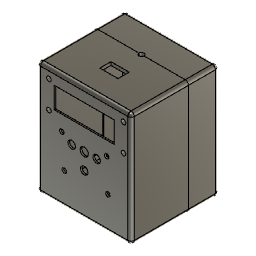
alarmClock (Autodesk Fusion 360 design; units mm, degrees)
Autodesk Fusion 360 part; units mm, degrees
sketch "Sketch1" plane through (0, 0, 0) normal (0, 0, 1) x (1, 0, 0)
  line L0 (35, 32.5) -> (-35, 32.5)
  line L1 (-35, 32.5) -> (-35, -32.5)
  line L2 (-35, -32.5) -> (35, -32.5)
  line L3 (35, -32.5) -> (35, 32.5)
  line L4 (35, 32.5) -> (-35, -32.5) construction
  line L5 (-35, 32.5) -> (35, -32.5) construction
  dimension "d6" = 70
  dimension "d7" = 65
  constraint horizontal L0
  constraint perpendicular L0 L1
  constraint parallel L0 L2
  constraint parallel L1 L3
  constraint coincident L4 origin
  constraint coincident L5 origin
  measures "d6" distance of L1.end L2.end
  measures "d7" distance of L0.end L1.end
extrude "Extrude1" add sketch "Sketch1" along normal blind 86 makes body 1
shell "Shell1" thickness 2.6 outward yes removed faces 0 bodies 1
sketch "Sketch2" plane through (0, 32.5, 0) normal (0, -1, 0) x (1, 0, 0)
  line L0 (-35, 0) -> (35, 0)
  line L1 (35, 0) -> (35, 86)
  line L2 (35, 86) -> (-35, 86)
  line L3 (-35, 86) -> (-35, 0)
  line L4 (28.1, 0) -> (19.9, 0)
  line L5 (19.9, 0) -> (19.9, 4.4)
  line L6 (19.9, 4.4) -> (28.1, 4.4)
  line L7 (28.1, 4.4) -> (28.1, 0)
  line L8 (24, 4.4) -> (24, 0) construction
  dimension "d11" = 8.2
  dimension "d12" = 4.4
  dimension "d13" = 11
  constraint horizontal L4
  constraint vertical L5
  constraint horizontal L6
  constraint vertical L7
  constraint coincident L0 L4.start
  constraint midpoint L6 L8.start
  constraint midpoint L4 L8.end
  measures "d11" distance of L5 L7
  measures "d12" distance of L4 L6
  measures "d13" distance of L1 L8
extrude "Extrude2" cut sketch "Sketch2" against normal up to surface (2.6 mm away) contours L0 L4 L5 L6 L7 bodies 1
sketch "Sketch3" plane through (0, 0, 0) normal (0, 0, 1) x (-1, 0, 0)
  line L0 (-35, 32.5) -> (-35, -32.5)
  line L1 (-35, -32.5) -> (-28.1, -32.5)
  line L2 (-28.1, -32.5) -> (-28.1, -35.1)
  line L3 (-28.1, -35.1) -> (-19.9, -35.1)
  line L4 (-19.9, -35.1) -> (-19.9, -32.5)
  line L5 (-19.9, -32.5) -> (35, -32.5)
  line L6 (35, -32.5) -> (35, 32.5)
  line L7 (35, 32.5) -> (-35, 32.5)
  line L8 (-24, -35.1) -> (-24, 32.5) construction
  line L9 (-16.6, -30.5) -> (-31.4, -30.5) construction
  line L10 (-31.4, -30.5) -> (-31.4, 10) construction
  line L11 (-31.4, 10) -> (-16.6, 10) construction
  line L12 (-16.6, 10) -> (-16.6, -30.5) construction
  circle A0 centre (-16.6, 10) radius 0.605
  circle A1 centre (-31.4, 10) radius 0.605
  circle A2 centre (-31.4, -30.5) radius 0.605
  circle A3 centre (-16.6, -30.5) radius 0.605
  line L13 (-31.4, 11.9) -> (-16.6, 11.9)
  line L14 (-16.6, 11.9) -> (-31.4, 11.9)
  line L15 (-31.4, 11.9) -> (-31.4, 13.3)
  line L16 (-31.4, 13.3) -> (-16.6, 13.3)
  line L17 (-16.6, 13.3) -> (-16.6, 11.9)
  line L18 (30.7, -26.5) -> (13, -26.5) construction
  line L19 (13, -26.5) -> (13, -0.8) construction
  line L20 (13, -0.8) -> (30.7, -0.8) construction
  line L21 (30.7, -0.8) -> (30.7, -26.5) construction
  circle A4 centre (13, -26.5) radius 1.5
  circle A5 centre (30.7, -26.5) radius 1.5
  circle A6 centre (30.7, -0.8) radius 1.5
  circle A7 centre (13, -0.8) radius 1.5
  line L22 (35, -10.8333) -> (-35, -10.8333) construction
  point P0 (-24, -30.5)
  dimension "d16" = 40.5
  dimension "d17" = 14.8
  dimension "d18" = 2
  dimension "d19" = 1.21
  dimension "d20" = 1.21
  dimension "d21" = 1.21
  dimension "d22" = 1.21
  dimension "d25" = -1.9
  dimension "d26" = 1.4
  dimension "d29" = 22
  dimension "d30" = 6
  dimension "d31" = 17.7
  dimension "d32" = 25.7
  dimension "d33" = 3
  dimension "d34" = 3
  dimension "d35" = 3
  dimension "d36" = 3
  dimension "d93" = 21.6667
  constraint midpoint L3 L8.start
  constraint coincident L7 L8.end
  constraint perpendicular L7 L8
  constraint horizontal L9
  constraint vertical L10
  constraint horizontal L11
  constraint vertical L12
  constraint midpoint L9 P0
  constraint coincident L8 P0
  constraint coincident L11.end L12.start
  constraint coincident L10.end L11.start
  constraint coincident L9.end L10.start
  constraint coincident L9.start L12.end
  constraint horizontal L14
  constraint vertical L15
  constraint horizontal L16
  constraint vertical L17
  constraint coincident L13.start L15
  constraint horizontal L18
  constraint vertical L19
  constraint horizontal L20
  constraint vertical L21
  constraint coincident L18.end L19.start
  constraint coincident L18.start L21.end
  constraint coincident L20.end L21.start
  constraint coincident L19.end L20.start
  constraint coincident L6 L22.start
  constraint coincident L0 L22.end
  constraint perpendicular L0 L22
  measures "d16" distance of L9 L11
  measures "d17" distance of L10 L12
  measures "d18" distance of L5 L9
  measures "d19" diameter of A0
  measures "d20" diameter of A1
  measures "d21" diameter of A2
  measures "d22" diameter of A3
  measures "d26" distance of L13 L16
  measures "d29" distance of L6 L19
  measures "d30" distance of L5 L18
  measures "d31" distance of L19 L21
  measures "d32" distance of L18 L20
  measures "d33" diameter of A7
  measures "d34" diameter of A6
  measures "d35" diameter of A5
  measures "d36" diameter of A4
  measures "d93" distance of L5 L22
extrude "Extrude5" cut sketch "Sketch3" against normal up to surface (2.6 mm away) contours A4 | A5 | A6 | A7 bodies 1
extrude "Extrude3" cut sketch "Sketch3" against normal up to surface (2.6 mm away) contours A0 | A1 | A2 | A3 bodies 1
extrude "Extrude4" add sketch "Sketch3" along normal blind 7.2 contours L13 L14 L15 L16 L17 bodies 1
chamfer "Chamfer2" distance 7 angle 45 1 edges at (24, -13.3, 0) on bodies 1
sketch "Sketch4" plane through (0, -32.5, 0) normal (0, 1, 0) x (-1, 0, 0)
  line L0 (-35, 0) -> (35, 0)
  line L1 (35, 0) -> (35, 86)
  line L2 (35, 86) -> (-35, 86)
  line L3 (-35, 86) -> (-35, 0)
  line L4 (0, 86) -> (0, 0) construction
  circle A0 centre (0, 31) radius 3
  circle A1 centre (0, 44) radius 3.3
  line L5 (-35, 44) -> (35, 44) construction
  circle A2 centre (10, 44) radius 3
  circle A3 centre (-10, 44) radius 3
  line L6 (10, 44) -> (18, 44) construction
  line L7 (18, 44) -> (18, 50) construction
  line L8 (18, 50) -> (10, 50) construction
  line L9 (10, 50) -> (10, 44) construction
  line L10 (-10, 44) -> (-18, 44) construction
  line L11 (-18, 44) -> (-18, 49) construction
  line L12 (-18, 49) -> (-10, 49) construction
  line L13 (-10, 49) -> (-10, 44) construction
  line L14 (18, 50) -> (19, 50) construction
  line L15 (19, 50) -> (19, 24) construction
  line L16 (19, 24) -> (18, 24) construction
  line L17 (18, 24) -> (18, 50) construction
  line L18 (-18, 49) -> (-16, 49) construction
  line L19 (-16, 49) -> (-16, 23) construction
  line L20 (-16, 23) -> (-18, 23) construction
  line L21 (-18, 23) -> (-18, 49) construction
  circle A4 centre (-16, 23) radius 1.8 construction
  circle A5 centre (19, 24) radius 1.8 construction
  circle A6 centre (18, 50) radius 1.8 construction
  circle A7 centre (-18, 49) radius 1.8 construction
  line L22 (26.1, 59.2) -> (-26.1, 59.2)
  line L23 (-26.1, 59.2) -> (-26.1, 80.2)
  line L24 (-26.1, 80.2) -> (26.1, 80.2)
  line L25 (26.1, 80.2) -> (26.1, 59.2)
  line L26 (26.1, 59.2) -> (-26.1, 80.2) construction
  line L27 (-26.1, 59.2) -> (26.1, 80.2) construction
  line L28 (-24.1, 78.2) -> (24.1, 78.2)
  line L29 (24.1, 78.2) -> (24.1, 61.2)
  line L30 (24.1, 61.2) -> (-24.1, 61.2)
  line L31 (-24.1, 61.2) -> (-24.1, 78.2)
  line L32 (31.5, 80.5) -> (31.5, 58.8) construction
  line L33 (31.5, 80.5) -> (31.5, 58.8) construction
  line L34 (31.5, 58.8) -> (-28.3, 58.8) construction
  line L35 (-28.3, 58.8) -> (-28.3, 80.5) construction
  line L36 (-28.3, 80.5) -> (31.5, 80.5) construction
  circle A8 centre (31.5, 80.5) radius 1.85 construction
  circle A9 centre (31.5, 58.8) radius 1.85 construction
  circle A10 centre (-28.3, 80.5) radius 1.85 construction
  circle A11 centre (-28.3, 58.8) radius 1.85 construction
  circle A12 centre (18, 49) radius 1.8
  circle A13 centre (16, 23) radius 1.8
  circle A14 centre (-18, 50) radius 1.8
  circle A15 centre (-19, 24) radius 1.8
  circle A16 centre (28.3, 58.8) radius 1.85
  circle A17 centre (28.3, 80.5) radius 1.85
  circle A18 centre (-31.5, 80.5) radius 1.85
  circle A19 centre (-31.5, 58.8) radius 1.85
  line L37 (28, 55) -> (-29, 55)
  line L38 (-29, 55) -> (-29, 18)
  line L39 (-29, 18) -> (28, 18)
  line L40 (28, 18) -> (28, 55)
  point P0 (0, 69.7)
  dimension "d39" = 31
  dimension "d40" = 13
  dimension "d41" = 10
  dimension "d42" = 10
  dimension "d43" = 6
  dimension "d44" = 6
  dimension "d45" = 6
  dimension "d46" = 6.6
  dimension "d47" = 8
  dimension "d48" = 6
  dimension "d49" = 8
  dimension "d50" = 5
  dimension "d51" = 26
  dimension "d52" = 1
  dimension "d53" = 2
  dimension "d54" = 26
  dimension "d55" = 3.6
  dimension "d56" = 3.6
  dimension "d57" = 3.6
  dimension "d58" = 3.6
  dimension "d59" = 52.2
  dimension "d60" = 21
  dimension "d61" = 15.2
  dimension "d62" = 2
  dimension "d63" = 5.4
  dimension "d64" = 0.3
  dimension "d65" = 0.4
  dimension "d66" = 2.2
  dimension "d67" = 3.7
  dimension "d68" = 3.7
  dimension "d69" = 3.7
  dimension "d70" = 3.7
  dimension "d125" = 5
  dimension "d126" = 10
  dimension "d127" = 10
  dimension "d128" = 5
  constraint midpoint L2 L4.start
  constraint coincident L4.end origin
  constraint coincident L4 A0.centre
  constraint coincident L4 A1.centre
  constraint coincident L3 L5.start
  constraint coincident L1 L5.end
  constraint perpendicular L1 L5
  constraint coincident A1.centre L5
  constraint coincident L5 A2.centre
  constraint coincident L5 A3.centre
  constraint horizontal L6
  constraint vertical L7
  constraint horizontal L8
  constraint vertical L9
  constraint coincident A2.centre L6.start
  constraint horizontal L10
  constraint vertical L11
  constraint horizontal L12
  constraint vertical L13
  constraint coincident A3.centre L10.start
  constraint horizontal L14
  constraint vertical L15
  constraint horizontal L16
  constraint vertical L17
  constraint horizontal L18
  constraint vertical L19
  constraint horizontal L20
  constraint vertical L21
  constraint coincident L19.end L20.start
  constraint coincident L15.end L16.start
  constraint coincident L7.end L8.start
  constraint coincident L11.end L12.start
  constraint horizontal L22
  constraint perpendicular L22 L23
  constraint parallel L22 L24
  constraint parallel L23 L25
  constraint coincident L26 P0
  constraint coincident L27 P0
  constraint coincident L4 P0
  constraint parallel L25 L32
  constraint perpendicular L33 L34
  constraint parallel L33 L35
  constraint parallel L34 L36
  constraint coincident L32.start L33.start
  constraint coincident L32.end L33.end
  constraint coincident L35.end L36.start
  constraint coincident L34.end L35.start
  constraint symmetric L4 A4 A13
  constraint symmetric L4 A5 A15
  constraint symmetric L4 A6 A14
  constraint symmetric L4 A7 A12
  constraint symmetric L4 A8 A18
  constraint symmetric L4 A9 A19
  constraint symmetric L4 A10 A17
  constraint symmetric L4 A11 A16
  constraint horizontal L37
  constraint vertical L38
  constraint horizontal L39
  constraint vertical L40
  measures "d39" distance of L4.end A0.centre
  measures "d40" distance of A0.centre A1.centre
  measures "d41" distance of A1.centre A3.centre
  measures "d42" distance of A1.centre A2.centre
  measures "d43" diameter of A3
  measures "d44" diameter of A2
  measures "d45" diameter of A0
  measures "d46" diameter of A1
  measures "d47" distance of A2.centre L6.end
  measures "d48" distance of A2.centre L8.end
  measures "d49" distance of L11 L13
  measures "d50" distance of L10 L12
  measures "d51" distance of L7.end L16.end
  measures "d52" distance of L15 L17
  measures "d53" distance of L11.end L18.end
  measures "d54" distance of L11.end L20.end
  measures "d55" diameter of A4
  measures "d56" diameter of A5
  measures "d57" diameter of A6
  measures "d58" diameter of A7
  measures "d59" distance of L23.end L24.end
  measures "d60" distance of L22.end L23.end
  measures "d61" distance of A1.centre L22
  measures "d63" distance of L25 L32
  measures "d64" distance of L24 L32.start
  measures "d65" distance of L22 L32.end
  measures "d66" distance of L23 L35
  measures "d67" diameter of A8
  measures "d68" diameter of A9
  measures "d69" diameter of A10
  measures "d70" diameter of A11
  measures "d125" distance of A14.centre L37
  measures "d126" distance of A15.centre L38
  measures "d127" distance of A12.centre L40
  measures "d128" distance of A13.centre L39
extrude "Extrude13" cut sketch "Sketch4" against normal blind 1.3 contours L37 L38 L39 L40 bodies 1
extrude "Extrude6" cut sketch "Sketch4" against normal up to surface (2.6 mm away) contours A0 | A1 | A2 | A3 | L22 L23 L24 L25 | L28 L29 L30 L31 | A12 | A13 | A14 | A15 | A16 | A17 | A18 | A19 bodies 1
extrude "Extrude7" add sketch "Sketch4" along normal blind 1.2 from surface at -2.6 contours L22 L23 L24 L25 bodies 1
sketch "Sketch5" plane through (0, 0, 86) normal (0, 0, -1) x (1, 0, 0)
  line L0 (35, -32.5) -> (35, 32.5)
  line L1 (35, 32.5) -> (-35, 32.5)
  line L2 (-35, 32.5) -> (-35, -32.5)
  line L3 (-35, -32.5) -> (35, -32.5)
  line L4 (-35, 10.8333) -> (35, 10.8333) construction
  line L5 (35, 10.8333) -> (35, -10.8333)
  line L6 (35, -10.8333) -> (-35, -10.8333) construction
  line L7 (-35, -10.8333) -> (-35, 10.8333)
  line L8 (0, 32.5) -> (0, -32.5) construction
  line L9 (7.3, 6.3833) -> (-7.3, 6.3833)
  line L10 (-7.3, 6.3833) -> (-7.3, 15.2833)
  line L11 (-7.3, 15.2833) -> (7.3, 15.2833)
  line L12 (7.3, 15.2833) -> (7.3, 6.3833)
  line L13 (7.3, 6.3833) -> (-7.3, 15.2833) construction
  line L14 (-7.3, 6.3833) -> (7.3, 15.2833) construction
  circle A0 centre (0, -10.8333) radius 2
  line L15 (-1.9, -14.9333) -> (1.9, -14.9333)
  line L16 (1.9, -14.9333) -> (1.9, -6.7333)
  line L17 (1.9, -6.7333) -> (-1.9, -6.7333)
  line L18 (-1.9, -6.7333) -> (-1.9, -14.9333)
  line L19 (-1.9, -14.9333) -> (1.9, -6.7333) construction
  line L20 (1.9, -14.9333) -> (-1.9, -6.7333) construction
  line L21 (-1.9, -6.7333) -> (1.9, -6.7333)
  line L22 (1.9, -6.7333) -> (1.9, -3.7333)
  line L23 (1.9, -3.7333) -> (-1.9, -3.7333)
  line L24 (-1.9, -3.7333) -> (-1.9, -6.7333)
  line L25 (-1.9, -14.9333) -> (1.9, -14.9333)
  line L26 (1.9, -14.9333) -> (1.9, -17.9333)
  line L27 (1.9, -17.9333) -> (-1.9, -17.9333)
  line L28 (-1.9, -17.9333) -> (-1.9, -14.9333)
  point P0 (0, 10.8333)
  point P1 (0, -10.8333)
  dimension "d76" = 21.6667
  dimension "d77" = 21.6667
  dimension "d78" = 14.6
  dimension "d79" = 8.9
  dimension "d80" = 4
  dimension "d83" = 3.8
  dimension "d84" = 8.2
  dimension "d85" = 3
  dimension "d86" = 3
  constraint horizontal L4
  constraint vertical L5
  constraint horizontal L6
  constraint vertical L7
  constraint coincident L0 L5.end
  constraint coincident L2 L4.start
  constraint midpoint L1 L8.start
  constraint midpoint L3 L8.end
  constraint horizontal L9
  constraint perpendicular L9 L10
  constraint parallel L9 L11
  constraint parallel L10 L12
  constraint coincident L13 P0
  constraint coincident L14 P0
  constraint midpoint L4 P0
  constraint midpoint L6 P1
  constraint horizontal L15
  constraint perpendicular L15 L16
  constraint parallel L15 L17
  constraint parallel L16 L18
  constraint coincident L19 P1
  constraint coincident L20 P1
  constraint coincident P1 A0.centre
  constraint horizontal L21
  constraint vertical L22
  constraint horizontal L23
  constraint vertical L24
  constraint collinear L16 L22
  constraint horizontal L25
  constraint vertical L26
  constraint horizontal L27
  constraint vertical L28
  constraint collinear L16 L26
  measures "d76" distance of L1 L4
  measures "d77" distance of L3 L6
  measures "d78" distance of L10.end L11.end
  measures "d79" distance of L9.end L10.end
  measures "d80" diameter of A0
  measures "d83" distance of L16.end L17.end
  measures "d84" distance of L15.end L16.end
  measures "d85" distance of L21 L23
  measures "d86" distance of L15 L27
extrude "Extrude9" add sketch "Sketch5" along normal blind 4.9 contours L17 L21 L22 L23 L24 | L15 L25 L26 L27 L28 bodies 1
extrude "Extrude8" cut sketch "Sketch5" against normal up to surface (2.6 mm away) contours L9 L10 L11 L12 | A0 L16 | A0 L16 L18 | A0 L18 bodies 1
extrude "Extrude10" add sketch "Sketch5" along normal blind 4 from surface at 4.9 contours A0 L16 L18 | A0 L16 L17 L18 L21 | A0 L15 L16 L18 L25 | L17 L21 L22 L23 L24 | L15 L25 L26 L27 L28 bodies 1
chamfer "Chamfer1" distance 8.8 angle 45 2 edges at (0, 17.9333, 86) (0, 3.7333, 86) on bodies 1
ref_plane "WorkPlane1" through (-35, 10.8333, 86) normal (0, 1, 0) x (-1, 0, 0)
split "Split1" by plane through (-35, 10.8333, 86) normal (0, 1, 0) bodies 1 makes body 2 at (6.6333, 35.1, 60.5333)
sketch "Sketch6" plane through (0, 10.8333, 0) normal (0, -1, 0) x (1, 0, 0)
  line L0 (37.6, -2.6) -> (37.6, 88.6)
  line L1 (37.6, 88.6) -> (2, 88.6)
  line L2 (2, 88.6) -> (2, 86)
  line L3 (2, 86) -> (35, 86)
  line L4 (35, 86) -> (35, 0)
  line L5 (35, 0) -> (-35, 0)
  line L6 (-35, 0) -> (-35, 86)
  line L7 (-35, 86) -> (-2, 86)
  line L8 (-2, 86) -> (-2, 88.6)
  line L9 (-37.6, 88.6) -> (-37.6, -2.6)
  line L10 (-37.6, -2.6) -> (37.6, -2.6)
  line L11 (-32, 87.48) -> (-5, 87.48)
  line L12 (-5, 87.48) -> (-5, -1.48)
  line L13 (-5, -1.48) -> (-32, -1.48)
  line L14 (-32, -1.48) -> (-32, 87.48)
  line L15 (5, 87.48) -> (32, 87.48)
  line L16 (32, 87.48) -> (32, -1.48)
  line L17 (32, -1.48) -> (5, -1.48)
  line L18 (5, -1.48) -> (5, 87.48)
  line L19 (-36.48, 83) -> (36.48, 83)
  line L20 (36.48, 83) -> (36.48, 3)
  line L21 (36.48, 3) -> (-36.48, 3)
  line L22 (-36.48, 3) -> (-36.48, 83)
  line L23 (-2, 88.6) -> (-37.6, 88.6)
  dimension "d94" = 3
  dimension "d95" = 3
  dimension "d96" = 3
  dimension "d97" = 3
  dimension "d102" = 3
  dimension "d103" = 3
  dimension "d110" = 1.48
  dimension "d111" = 1.48
  dimension "d112" = 1.48
  dimension "d113" = 1.48
  constraint horizontal L11
  constraint vertical L12
  constraint horizontal L13
  constraint vertical L14
  constraint horizontal L15
  constraint vertical L16
  constraint horizontal L17
  constraint vertical L18
  constraint horizontal L19
  constraint vertical L20
  constraint horizontal L21
  constraint vertical L22
  constraint collinear L13 L17
  constraint collinear L11 L15
  measures "d94" distance of L3.end L16
  measures "d95" distance of L2 L18
  measures "d96" distance of L8 L12
  measures "d97" distance of L6 L14
  measures "d102" distance of L5 L21
  measures "d103" distance of L3 L19
  measures "d110" distance of L3 L15
  measures "d111" distance of L5 L17
  measures "d112" distance of L4 L20
  measures "d113" distance of L6 L22
extrude "Extrude11" cut sketch "Sketch6" against normal blind 4.8 contours L3 L15 L16 L18 | L7 L11 L12 L14 | L4 L19 L20 L21 | L5 L16 L17 L18 | L5 L12 L13 L14 | L6 L19 L21 L22 bodies 2
sketch "Sketch8" plane through (0, 10.8333, 0) normal (0, 1, 0) x (-1, 0, 0)
  line L0 (5, 87.48) -> (5, -1.48)
  line L1 (5, -1.48) -> (32, -1.48)
  line L2 (32, -1.48) -> (32, 87.48)
  line L3 (-36.48, 3) -> (36.48, 3)
  line L4 (36.48, 3) -> (36.48, 83)
  line L5 (-32, -1.48) -> (-5, -1.48)
  line L6 (-5, -1.48) -> (-5, 87.48)
  line L7 (-32, 87.48) -> (-32, -1.48)
  line L8 (-36.48, 83) -> (-36.48, 3)
  line L9 (32, 87.48) -> (5, 87.48)
  line L10 (36.48, 83) -> (-36.48, 83)
  line L11 (-5, 87.48) -> (-32, 87.48)
  line L12 (31.64, -1.12) -> (31.64, 87.12)
  line L13 (31.64, 87.12) -> (5.36, 87.12)
  line L14 (5.36, 87.12) -> (5.36, -1.12)
  line L15 (5.36, -1.12) -> (31.64, -1.12)
  line L16 (-36.12, 82.64) -> (-36.12, 3.36)
  line L17 (-36.12, 3.36) -> (36.12, 3.36)
  line L18 (36.12, 3.36) -> (36.12, 82.64)
  line L19 (36.12, 82.64) -> (-36.12, 82.64)
  line L20 (-37.6, 88.6) -> (-37.6, -2.6)
  line L21 (-37.6, -2.6) -> (37.6, -2.6)
  line L22 (37.6, -2.6) -> (37.6, 88.6)
  line L23 (37.6, 88.6) -> (2, 88.6)
  line L24 (2, 88.6) -> (2, 86)
  line L25 (2, 86) -> (35, 86)
  line L26 (35, 86) -> (35, 0)
  line L27 (35, 0) -> (-35, 0)
  line L28 (-35, 0) -> (-35, 86)
  line L29 (-35, 86) -> (-2, 86)
  line L30 (-2, 86) -> (-2, 88.6)
  line L31 (-2, 88.6) -> (-37.6, 88.6)
extrude "Extrude12" add sketch "Sketch8" along normal blind 4 contours L12 L13 L14 L25 | L6 L7 L11 L29 | L17 L18 L19 L26 | L16 L17 L19 L28 | L12 L14 L15 L27 | L5 L6 L7 L27 bodies 1
fillet "Fillet3" radius 2.6 12 edges at (0, -35.1, -2.6) (-37.6, -35.1, 43) (-37.6, 0, -2.6) (-37.6, 35.1, 43) (37.6, -35.1, 43) (37.6, 0, -2.6) (0, 35.1, -2.6) (-37.6, 0, 88.6) (0, -35.1, 88.6) (37.6, 0, 88.6) (0, 35.1, 88.6) (37.6, 35.1, 43) on bodies 1 2
fillet "Fillet1" radius 2 8 edges at (0, -32.5, 86) (35, -32.5, 43) (0, -32.5, 0) (-35, -32.5, 43) (-35, -10.8333, 0) (35, -10.8333, 0) (35, -10.8333, 86) (-35, -10.8333, 86) on bodies 1
fillet "Fillet2" radius 2 7 edges at (35, 32.5, 43) (35, 21.6667, 86) (-35, 21.6667, 86) (-35, 32.5, 43) (0, 32.5, 86) (35, 21.6667, 0) (-35, 21.6667, 0) on bodies 2
equation "innerWidth = 70 mm"
equation "shellThickness = 2.6 mm"
equation "innerLength = 65 mm"
equation "innerHeight = 86 mm"
equation "d6 = innerWidth"
equation "d7 = innerLength"
equation "d8 = innerHeight"
equation "d10 = shellThickness"
equation "d76 = innerLength / 3"
equation "d77 = innerLength / 3"
equation "d93 = innerLength / 3"
equation "connectorLength = 4 mm"
equation "connectorClearance = 0.36 mm"
equation "d108 = -connectorLength - 0.8 mm"
equation "d110 = ( connectorClearance / 2 ) + ( shellThickness / 2 )"
equation "d111 = ( connectorClearance / 2 ) + ( shellThickness / 2 )"
equation "d112 = ( connectorClearance / 2 ) + ( shellThickness / 2 )"
equation "d113 = ( connectorClearance / 2 ) + ( shellThickness / 2 )"
equation "d114 = -connectorClearance"
equation "d115 = -connectorClearance"
equation "d116 = connectorLength"
equation "d129 = -( shellThickness / 2 )"
named bodies: "front", "back"
